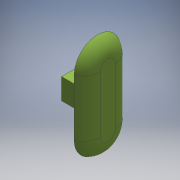
# Autodesk Inventor part: ET18
Saved by Autodesk Inventor 2016 (Build 200138000, 138)
## iProperties
Created: 2016-03-28
Part Number: ET18
Material: Genérico
Document SubType Name: Modeling
Designer: Usuario1
Density: 1 g/cm^3
Appearance: Valor por defecto
Author: Usuario1
Autodesk Inventor part; units mm, degrees
ref_plane "YZ Plane" through (0, 0, 0) normal (1, 0, 0) x (0, 1, 0)
ref_plane "XZ Plane" through (0, 0, 0) normal (0, 1, 0) x (-1, 0, 0)
ref_plane "XY Plane" through (0, 0, 0) normal (0, 0, 1) x (1, 0, 0)
sketch "Boceto1" plane through (0, 0, 0) normal (1, 0, 0) x (0, 1, 0)
  circle A0 centre (0, 0) radius 1.0926
  circle A1 centre (-0.389, 0.0377) radius 0.6841
  line L0 (-0.2217, -0.7829) -> (-0.172, -0.9902)
  line L1 (0.4827, -0.8628) -> (0.4482, -0.6469)
  arc A2 (0.4827, -0.8628) -> (-0.172, -0.9902) centre (0.3728, -2.0444) ccw
  arc A3 (-0.2217, -0.7829) -> (-0.0098, -0.6943) centre (-0.3611, -0.1519) ccw
  arc A4 (0.2046, -0.6494) -> (-0.0098, -0.6943) centre (0.1354, -0.8536) ccw
  arc A5 (0.2046, -0.6494) -> (0.4482, -0.6469) centre (0.3201, -0.0382) ccw
  line L2 (0.623, 0.1405) -> (0.623, -0.1283)
  line L3 (0.8433, -0.1283) -> (0.8433, 0.1405)
  arc A6 (0.8433, 0.1405) -> (0.623, 0.1405) centre (0.7332, 0.1405) ccw
  arc A7 (0.623, -0.1283) -> (0.8433, -0.1283) centre (0.7332, -0.1283) ccw
  line L4 (0.48, 0.6571) -> (0.5054, 0.8687)
  line L5 (-0.1528, 0.9768) -> (-0.1954, 0.7624)
  arc A8 (-0.1528, 0.9768) -> (0.5054, 0.8687) centre (0.3609, 2.0465) ccw
  arc A9 (0.48, 0.6571) -> (0.2505, 0.6476) centre (0.3914, 0.0169) ccw
  arc A10 (0.0338, 0.6801) -> (0.2505, 0.6476) centre (0.1696, 0.8475) ccw
  arc A11 (0.0338, 0.6801) -> (-0.1954, 0.7624) centre (-0.2869, 0.147) ccw
  circle A12 centre (0, 0) radius 1.1994
  constraints: 20 point on circle, 13 centre point, 12 end point, 1 coincident
extrude "Extrusión1" add sketch "Boceto1" along normal blind 0.05 contours A6 L3 A7 L2
fillet "Empalme1" radius 0.08 4 edges at (0.05, 0.7332, 0.2507) (0.05, 0.623, 0.0061) (0.05, 0.7332, -0.2385) (0.05, 0.8433, 0.0061)
sketch "Boceto2" plane through (0, 0, 0) normal (-1, 0, 0) x (0, 0, 1)
  circle A0 centre (-0.7722, -0.6284) radius 0.0625
  circle A1 centre (0.7346, -0.6284) radius 0.0625
  circle A2 centre (0.0033, 1.0028) radius 0.0698
  line L0 (-0.713, 0.203) -> (-0.713, 0.103)
  line L1 (-0.713, 0.103) -> (-0.813, 0.103)
  line L2 (-0.813, 0.103) -> (-0.813, 0.203)
  line L3 (-0.813, 0.203) -> (-0.713, 0.203)
  line L4 (0.0439, 0.7832) -> (0.0439, 0.6832)
  line L5 (0.0439, 0.6832) -> (-0.0561, 0.6832)
  line L6 (-0.0561, 0.6832) -> (-0.0561, 0.7832)
  line L7 (-0.0561, 0.7832) -> (0.0439, 0.7832)
  line L8 (0.825, 0.1653) -> (0.825, 0.0653)
  line L9 (0.825, 0.0653) -> (0.725, 0.0653)
  line L10 (0.725, 0.0653) -> (0.725, 0.1653)
  line L11 (0.725, 0.1653) -> (0.825, 0.1653)
  line L12 (0.0623, -0.289) -> (0.0623, -0.489)
  line L13 (0.0623, -0.489) -> (-0.1377, -0.489)
  line L14 (-0.1377, -0.489) -> (-0.1377, -0.289)
  line L15 (-0.1377, -0.289) -> (0.0623, -0.289)
  circle A3 centre (0, 0) radius 1.0926
  constraints: 32 end point, 4 centre point
extrude "Extrusión2" add sketch "Boceto2" along normal blind 0.12 contours L4 L5 L6 L7
